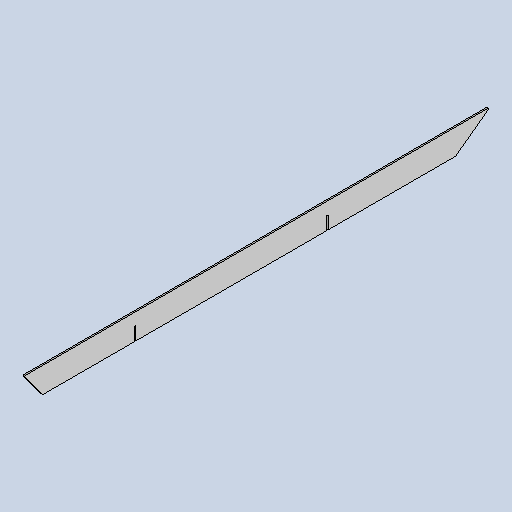
# Autodesk Inventor part: MSC 010.5 stringer cone
Saved by Autodesk Inventor 2025 (Build 290162010, 162A)
## iProperties
Created: 2024-06-26
Part Number: MSC 010.5 stringer cone
Material: Stainless Steel
Document SubType Name: Sheet Metal
Designer: pokla
Density: 8 g/cm^3
Sheet Metal Rule: AISI304 3mm Die 32
Appearance: Default
Stock Number: МОО 010.5 стрингер конус
Author: pokla
Autodesk Inventor part; units mm, degrees
ref_plane "YZ Plane" through (0, 0, 0) normal (1, 0, 0) x (0, 1, 0)
ref_plane "XZ Plane" through (0, 0, 0) normal (0, 1, 0) x (-1, 0, 0)
ref_plane "XY Plane" through (0, 0, 0) normal (0, 0, 1) x (1, 0, 0)
sketch "Sketch2" plane through (0, 0, 0) normal (1, 0, 0) x (0, 1, 0)
  line L0 (0, 0) -> (920, 0)
  line L1 (920, 0) -> (920, -50)
  line L2 (920, -50) -> (0, -50)
  line L3 (0, -50) -> (0, 0)
  line L4 (920, -50) -> (883.2713, 0) construction
  line L5 (920, 0) -> (851.9332, -50)
  line L6 (0, 0) -> (36.7287, -50)
  dimension "d28" = 920
  dimension "d29" = 50
  dimension "d31" = 36.3
  dimension "d32" = 53.7
  dimension "d36" = 53.7
  measures "d28" distance of L1.end L2.end
  measures "d29" distance of L0.end L1.end
  measures "d31" angle of L1 L4
  measures "d32" angle of L5 L1
  measures "d36" angle of L0 L6
extrude "Plate2" add sketch "Sketch2" along normal blind 3 contours L0 L5 L2 L6
chamfer "Corner Chamfer1" distance 3 angle 45 2 edges at (1.5, 920, 0) (1.5, 0, 0)
fillet "Corner Round1" radius 6 2 edges at (1.5, 36.7287, -50) (1.5, 851.9332, -50)
sketch "Sketch3" plane through (3, 0, 0) normal (1, 0, 0) x (0, 0, -1)
  line L0 (24, 217.54) -> (50, 217.54)
  line L1 (50, 217.54) -> (50, 220.54)
  line L2 (50, 220.54) -> (24, 220.54)
  line L3 (24, 220.54) -> (24, 217.54)
  line L4 (50, 849.9663) -> (50, 39.766) projected
  line L5 (50, 219.04) -> (0, 219.04) construction
  line L6 (0, 3) -> (0, 917) projected
  line L7 (50, 599.04) -> (0, 599.04) construction
  line L8 (24, 597.54) -> (50, 597.54)
  line L9 (50, 597.54) -> (50, 600.54)
  line L10 (50, 600.54) -> (24, 600.54)
  line L11 (24, 600.54) -> (24, 597.54)
  point P0 (0, 0)
  dimension "d39" = 26
  dimension "d40" = 3
  dimension "d41" = 219.04
  dimension "d42" = 599.04
  dimension "d43" = 3
  dimension "d44" = 26
  constraints: 20 end point, 4 parallel, 4 point on line, 3 horizontal, 3 perpendicular, 2 midpoint
  measures "d39" distance of L2.end L1.end
  measures "d40" distance of L0.end L1.end
  measures "d41" distance from line of point (0, 0) L5
  measures "d42" distance from line of point (0, 0) L7
  measures "d43" distance of L8.end L9.end
  measures "d44" distance of L9.end L10.end
extrude "Extrusion1" cut sketch "Sketch3" against normal through all
equation "\"d36\" = d32"
equation "\"d40\" = Thickness"
equation "\"d43\" = Thickness"
equation "\"d44\" = d39"
equation "\"d30\" = Thickness"
equation "\"BendReliefWidth\" = Thickness"
equation "\"BendReliefDepth\" = 0.5 * Thickness"
equation "\"CornerReliefSize\" = 4 * Thickness"
equation "\"MinimumRemnant\" = 2 * Thickness"
equation "\"TransitionRadius\" = BendRadius"
equation "\"JacobiRadiusSize\" = BendRadius"
equation "\"GapSize\" = Thickness"
equation "\"Thickness\" = 3"
equation "\"BendRadius\" = 5"
body "Solid2"
